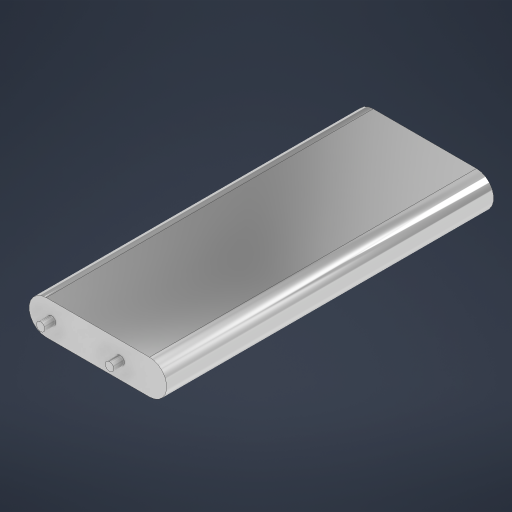
# Autodesk Inventor part: battery
Saved by Autodesk Inventor 2023 (Build 270158000, 158)
## iProperties
Created: 2023-12-07
Part Number: battery
Material: Generic
Document SubType Name: Modeling
Designer: Andi
Density: 1 g/cm^3
Appearance: Chrome - Polished
Author: Andi
Autodesk Inventor part; units mm, degrees
ref_plane "YZ Plane" through (0, 0, 0) normal (1, 0, 0) x (0, 1, 0)
ref_plane "XZ Plane" through (0, 0, 0) normal (0, 1, 0) x (-1, 0, 0)
ref_plane "XY Plane" through (0, 0, 0) normal (0, 0, 1) x (1, 0, 0)
sketch "Sketch1" plane through (0, 0, 0) normal (0, 0, 1) x (1, 0, 0)
  line L0 (-6, 0) -> (6, 0) construction
  line L1 (-6, -2) -> (6, -2)
  line L2 (6, 2) -> (-6, 2)
  arc A0 (-6, 2) -> (-6, -2) centre (-6, 0) ccw
  arc A1 (6, -2) -> (6, 2) centre (6, 0) ccw
  point P0 (0, 0)
  point P1 (0, 0)
  point P2 (-8, 0)
  point P3 (8, 0)
  dimension "d0" = 4
  dimension "d1" = 16
  constraints: 8 end point, 6 point on circle, 4 tangent, 2 centre point, 1 coincident, 1 horizontal, 1 midpoint, 1 parallel
  measures "d0" distance between parallel lines of L1 L2
  measures "d1" distance of point (-8, 0) point (8, 0)
extrude "Extrusion1" add sketch "Sketch1" along normal mid plane 38
sketch "Sketch2" plane through (0, 0, 19) normal (0, 0, 1) x (1, 0, 0)
  circle A0 centre (2.5947, 0) radius 0.5
  circle A1 centre (-5.4053, 0) radius 0.5
  point P0 (0, 0)
  dimension "d4" = 8
  dimension "d5" = 1
  constraints: 2 centre point, 1 equal radius, 1 horizontal alignment
  measures "d4" distance of A1.centre A0.centre
  measures "d5" diameter of A0
extrude "Extrusion2" add sketch "Sketch2" along normal blind 1.25
body "Solid1"
